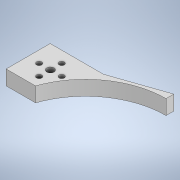
# Autodesk Inventor part: NewShooterFlicker
Saved by Autodesk Inventor 2020 (Build 240168000, 168)
## iProperties
Created: 2021-04-22
Part Number: NewShooterFlicker
Material: Generic
Document SubType Name: Modeling
Designer: tdmp4
Density: 1 g/cm^3
Appearance: Default
Author: tdmp4
Autodesk Inventor part; units mm, degrees
ref_plane "YZ Plane" through (0, 0, 0) normal (1, 0, 0) x (0, 1, 0)
ref_plane "XZ Plane" through (0, 0, 0) normal (0, 1, 0) x (-1, 0, 0)
ref_plane "XY Plane" through (0, 0, 0) normal (0, 0, 1) x (1, 0, 0)
sketch "Sketch1" plane through (0, 0, 0) normal (0, 1, 0) x (-1, 0, 0)
  arc A0 (0, -69.85) -> (65.9911, -22.8953) centre (0, 0) ccw
  line L0 (0, 0) -> (60.4919, -34.925)
  line L1 (0, 0) -> (69.85, 0) construction
  line L2 (60.4919, -34.925) -> (82.4889, -47.625)
  line L3 (60.4919, -34.925) -> (71.4904, -41.275)
  line L4 (60.4919, -34.925) -> (60.4919, -47.625)
  line L5 (60.4919, -47.625) -> (82.4889, -47.625)
  line L6 (60.4919, -34.925) -> (82.4889, -34.925)
  line L7 (82.4889, -34.925) -> (82.4889, -47.625)
  line L8 (82.4889, -34.925) -> (60.4919, -47.625)
  circle A1 centre (71.4904, -41.275) radius 9.779
  circle A2 centre (71.4904, -41.275) radius 3.175
  circle A3 centre (71.4904, -51.054) radius 2.286
  circle A4 centre (71.4904, -31.496) radius 2.286
  circle A5 centre (81.2694, -41.275) radius 2.286
  circle A6 centre (61.7114, -41.275) radius 2.286
  line L9 (65.9911, -22.8953) -> (91.3911, -22.8953)
  line L10 (91.3911, -22.8953) -> (91.3911, -60.9953)
  line L11 (91.3911, -60.9953) -> (33.2947, -60.9953)
  line L12 (0, 0) -> (0, -69.85)
  line L13 (0, 0) -> (65.9911, -22.8953)
  line L14 (0, -69.85) -> (0, -76.585)
  line L15 (0, -76.585) -> (45.4402, -60.9953)
  dimension "d0" = 139.7
  dimension "d1" = 30
  dimension "d2" = 25.4
  dimension "d3" = 19.558
  dimension "d4" = 6.35
  dimension "d5" = 4.572
  dimension "d6" = 4.572
  dimension "d7" = 4.572
  dimension "d8" = 4.572
  dimension "d9" = 25.4
  dimension "d10" = 38.1
  constraints: 32 end point, 7 centre point, 7 point on circle, 4 perpendicular, 3 coincident, 3 horizontal, 3 vertical, 1 equal length, 1 midpoint, 1 point on line
  measures "d0" diameter of A0
  measures "d1" angle of L0 L1
  measures "d2" distance of L0.end L2.end
  measures "d3" diameter of A1
  measures "d4" diameter of A2
  measures "d5" diameter of A3
  measures "d6" diameter of A4
  measures "d7" diameter of A5
  measures "d8" diameter of A6
  measures "d9" distance of L9.start L9.end
  measures "d10" distance of L9.end L10.end
extrude "Extrusion1" add sketch "Sketch1" along normal blind 12.7 contours A0 L9 L10 L11 | L6 A1 L2 | L2 A1 A6 L4 | L11 L15 L14 A0 | A1 L6 L8 A2 L2 | L2 A2 L8 A1 A6 | A1 A4 L6 | A6 A1 L8 L4 | L6 L8 A1 | L8 A1 A5 L2 A2 | A2 L2 A1 L5 L8 | L8 A1 L5 | L7 A5 A1 L8 | L5 A1 A3 | A1 A5 L7 L2 | L2 L5 A1
body "Solid1"
